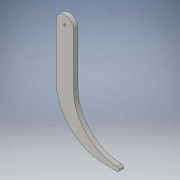
# Autodesk Inventor part: Bottom IntakeBar
Saved by Autodesk Inventor 2016 (Build 200138000, 138)
## iProperties
Created: 2016-01-16
Part Number: Bottom IntakeBar
Material: Generic
Document SubType Name: Modeling
Designer: Mentor1102
Density: 1 g/cm^3
Appearance: Default
Author: Mentor1102
Autodesk Inventor part; units mm, degrees
ref_plane "YZ Plane" through (0, 0, 0) normal (1, 0, 0) x (0, 1, 0)
ref_plane "XZ Plane" through (0, 0, 0) normal (0, 1, 0) x (-1, 0, 0)
ref_plane "XY Plane" through (0, 0, 0) normal (0, 0, 1) x (1, 0, 0)
sketch "Sketch1" plane through (0, 0, 0) normal (0, 0, 1) x (1, 0, 0)
  circle A0 centre (-132.0723, 175.8198) radius 3.175
  arc A1 (-106.6723, 175.8198) -> (-157.4723, 175.8198) centre (-132.0723, 175.8198) ccw
  arc A2 (-106.6723, 23.4198) -> (20.3277, -103.5802) centre (20.3277, 23.4198) ccw
  arc A3 (-157.4723, 23.4198) -> (-17.7723, -116.2802) centre (-17.7723, 23.4198) ccw
  line L0 (-157.4723, 175.8198) -> (-157.4723, 23.4198)
  line L1 (-106.6723, 23.4198) -> (-106.6723, 175.8198)
  line L2 (-17.7723, -116.2802) -> (20.3277, -116.2802)
  arc A4 (20.3277, -116.2802) -> (20.3277, -103.5802) centre (20.3277, -109.9302) ccw
  dimension "d23" = 6.35
  dimension "d24" = 50.8
  dimension "d25" = 25.4
  dimension "d26" = 127
  dimension "d27" = 139.7
  dimension "d28" = 152.4
  dimension "d29" = 152.4
  dimension "d30" = 6.35
  dimension "d31" = 38.1
  constraints: 8 point on circle, 6 end point, 5 centre point, 3 tangent, 1 horizontal, 1 parallel, 1 vertical
  measures "d23" diameter of A0
  measures "d24" distance between parallel lines of L1 L0
  measures "d25" radius of A1
  measures "d26" radius of A2
  measures "d27" radius of A3
  measures "d28" distance of L1.start L1.end
  measures "d29" distance of L0.start L0.end
  measures "d30" radius of A4
  measures "d31" distance of L2.start L2.end
extrude "Extrusion2" add sketch "Sketch1" along normal blind 12.7
body "Solid2"
